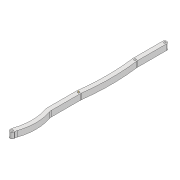
# Autodesk Inventor part: Part_7
Saved by Autodesk Inventor 2022 (Build 260153000, 153)
## iProperties
Created: 2022-04-26
Part Number: Part_7
Material: Generic
Document SubType Name: Modeling
Designer: dell
Density: 1 g/cm^3
Appearance: Default
Author: dell
Autodesk Inventor part; units mm, degrees
ref_plane "YZ Plane" through (0, 0, 0) normal (1, 0, 0) x (0, 1, 0)
ref_plane "XZ Plane" through (0, 0, 0) normal (0, 1, 0) x (-1, 0, 0)
ref_plane "XY Plane" through (0, 0, 0) normal (0, 0, 1) x (1, 0, 0)
sketch "Sketch1" plane through (0, 0, 0) normal (0, 1, 0) x (-1, 0, 0)
  line L0 (0, 0) -> (0, -212.9) construction
  line L1 (-3, 0) -> (-3, -212.9)
  line L2 (3, -212.9) -> (3, 0)
  arc A0 (3, 0) -> (-3, 0) centre (0, 0) ccw
  arc A1 (-3, -212.9) -> (3, -212.9) centre (0, -212.9) ccw
  circle A2 centre (0, 0) radius 1.5
  circle A3 centre (0, -212.9) radius 1.5
  circle A4 centre (0, -171.332) radius 1.5
  circle A5 centre (0, -92.628) radius 1.5
  arc A6 (3, -92.628) -> (3, -171.332) centre (300.4078, -131.98) ccw
  arc A7 (-3, -92.628) -> (-3, -171.332) centre (294.4078, -131.98) ccw
  arc A8 (3, -2) -> (3, -50) centre (68.7571, -26) ccw
  arc A9 (-3, -2) -> (-3, -50) centre (62.7571, -26) ccw
  point P0 (0, -106.45)
  dimension "d0" = 212.9
  dimension "d1" = 6
  dimension "d2" = 3
  dimension "d3" = 3
  dimension "d6" = 3
  dimension "d7" = 171.332
  dimension "d8" = 3
  dimension "d9" = 92.628
  dimension "d10" = 300
  dimension "d11" = 300
  dimension "d14" = 2
  dimension "d15" = 50
  dimension "d16" = 70
  dimension "d17" = 70
  constraints: 12 point on circle, 10 centre point, 10 point on line, 8 end point, 6 horizontal alignment, 4 tangent, 2 coincident, 1 midpoint, 1 parallel, 1 vertical
  measures "d0" distance of L0.start L0.end
  measures "d1" diameter of A1
  measures "d2" diameter of A2
  measures "d3" diameter of A3
  measures "d6" diameter of A4
  measures "d7" distance of L0.start A4.centre
  measures "d8" diameter of A5
  measures "d9" distance of L0.start A5.centre
  measures "d10" radius of A6
  measures "d11" radius of A7
  measures "d14" vertical distance of L0.start A8.start
  measures "d15" vertical distance of L0.start A8.end
  measures "d16" radius of A8
  measures "d17" radius of A9
extrude "Extrusion1" add sketch "Sketch1" along normal blind 8 contours A0 L2 A8 A6 A1 L1 | L1 A9 | L1 A7
fillet "Fillet1" radius 10 8 edges at (-3, 4, -2) (3, 4, -2) (3, 4, -50) (-3, 4, -50) (-3, 4, -92.628) (-3, 4, -171.332) (3, 4, -92.628) (3, 4, -171.332)
body "Solid1"
